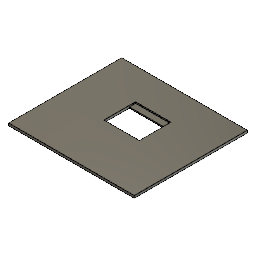
front _oledv1 (Autodesk Fusion 360 design; units mm, degrees)
Autodesk Fusion 360 part; units mm, degrees
box "BoxPrimitive1" add length 90 width 100 height 2 placed x (0, 0, 1) y (1, 0, 0) z (0, 1, 0) at (0, 0, -10)
box "BoxPrimitive2" cut length 20 width 28 height -10 placed x (0, 0, -1) y (-1, 0, 0) z (0, 1, 0) at (64, 2, 40)
box "BoxPrimitive3" cut length 5 width 28 height -1 placed x (0, 0, -1) y (-1, 0, 0) z (0, 1, 0) at (64, 2, 20)
